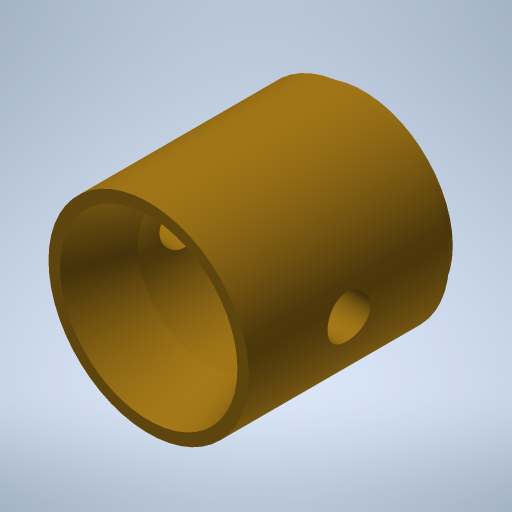
# Autodesk Inventor part: DLM-011
Saved by Autodesk Inventor 2024 (Build 280153000, 153)
## iProperties
Created: 2004-03-28
Part Number: DLM-011
Material: CuZn40
Description: Kolben
Document SubType Name: Modellieren
Designer: UR
Density: 1 g/cm^3
Appearance: Metall - Messing
Shininess: 20.0
Angle Display Precision: 2
Document Length Units: 11269
Document Angle Units: 11279
Document Time Units: 11290
Document Mass Units: 11283
Document Length Units Precision: 3
Document Angle Units Precision: 2
Density: 0.0
Volumn: 0.0
Area: 0.0
PropertySet Name: Model Information
Control State: 0
Master: False
Checked Out: False
Author: UR
Autodesk Inventor part; units mm, degrees
ref_plane "YZ Ebene" through (0, 0, 0) normal (1, 0, 0) x (0, 1, 0)
sketch "Skizze1" plane through (0, 0, 0) normal (0, 0, 1) x (1, 0, 0)
  line L0 (-3.068, 6.1973) -> (-3.068, 20.1973)
  line L1 (-3.068, 20.1973) -> (-2.318, 20.1973)
  line L2 (-2.318, 20.1973) -> (-2.318, 21.1973)
  line L3 (-2.318, 21.1973) -> (3.932, 21.1973)
  line L4 (-2.268, 6.1973) -> (-0.818, 10.1811)
  line L5 (-0.818, 10.1811) -> (-0.818, 17.1973)
  line L6 (-0.818, 17.1973) -> (3.932, 20.0514)
  line L7 (3.932, 20.0514) -> (3.932, 21.1973)
  line L8 (-2.268, 6.1973) -> (-3.068, 6.1973)
  dimension "d0" = 12.5
  dimension "d1" = 9.5
  dimension "d2" = 14
  dimension "d3" = 12.4
  dimension "d4" = 1
  dimension "d6" = 20
  dimension "d7" = 59
  dimension "d8" = 11
  dimension "d9" = 15
  constraints: 18 end point, 3 parallel, 3 perpendicular, 1 vertical
  measures "d0" diameter of L2 L7
  measures "d1" diameter of L5 L7
  measures "d2" diameter of L0 L7
  measures "d3" diameter of L4.start L7
  measures "d4" distance from line of L0.end L3
  measures "d6" angle of L5 L4
  measures "d7" angle of L7 L6
  measures "d8" distance from line of L8 L5.end
  measures "d9" distance between parallel lines of L8 L3
revolve "Drehung1" add sketch "Skizze1" angle 360 about axis through (3.932, 20.0514, 0) along (0, 1, 0)
ref_plane "Arbeitsebene1" through (10.932, 13.1973, 0) normal (1, 0, 0) x (0, 1, 0)
sketch "Skizze2" plane through (10.932, 13.1973, 0) normal (1, 0, 0) x (0, 1, 0)
  line L0 (-7, -7) -> (-7, 7) projected
  point P0 (0, 0)
  dimension "d13" = 7
  measures "d13" distance from line of point (0, 0) L0
ref_plane "Mittelebene" through (3.932, 13.1973, 0) normal (1, 0, 0) x (0, 1, 0)
hole "Bohrung1" at (10.932, 13.1973, 0) direction (-1, 0, 0) diameter 3 end through all
equation "\"d12\" = -0.5 * d2"
